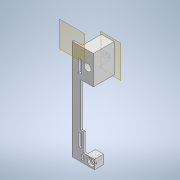
# Autodesk Inventor part: Display_Cover
Saved by Autodesk Inventor 2021 (Build 250183000, 183)
## iProperties
Created: 2020-08-10
Part Number: Display_Cover
Material: Generic
Document SubType Name: Modeling
Designer: ridvansong
Density: 1 g/cm^3
Appearance: Default
Author: ridvansong
Autodesk Inventor part; units mm, degrees
ref_plane "YZ Plane" through (0, 0, 0) normal (1, 0, 0) x (0, 1, 0)
ref_plane "XZ Plane" through (0, 0, 0) normal (0, 1, 0) x (-1, 0, 0)
ref_plane "XY Plane" through (0, 0, 0) normal (0, 0, 1) x (1, 0, 0)
ref_plane "Work Plane1" through (0, 0, 0) normal (0, 0, 1) x (1, 0, 0)
sketch "Sketch1" plane through (0, 0, 0) normal (0, 0, 1) x (1, 0, 0)
  line L0 (11.775, 18.625) -> (-4.025, 18.625) projected
  line L1 (11.775, 43.875) -> (11.775, 18.625) projected
  line L2 (-4.025, 43.875) -> (11.775, 43.875) projected
  line L3 (-4.025, 18.625) -> (-4.025, 43.875) projected
  line L4 (7.775, 43.875) -> (7.775, -42.625) projected
  line L5 (-4.025, 18.625) -> (6.775, 18.625)
  line L6 (6.775, 18.625) -> (6.775, 43.375)
  line L7 (6.775, 43.375) -> (-4.025, 43.375)
  line L8 (-4.025, 43.375) -> (-4.025, 18.625)
  circle A0 centre (1.775, 30.625) radius 1.3 projected
  line L9 (11.775, -42.625) -> (11.775, -34.625) projected
  line L10 (11.775, -34.625) -> (2.775, -34.625) projected
  line L11 (2.775, -34.625) -> (2.775, -42.625) projected
  line L12 (11.775, -42.625) -> (2.775, -42.625) projected
  line L13 (7.275, -34.625) -> (0.775, -34.625)
  line L14 (0.775, -34.625) -> (0.775, -42.125)
  line L15 (0.775, -42.125) -> (7.275, -42.125)
  line L16 (7.275, -42.125) -> (7.275, -34.625)
  circle A1 centre (4.775, -38.375) radius 1.3 projected
  point P0 (0, 0)
  point P1 (-4.025, 43.375)
  dimension "d0" = 0.5
  dimension "d1" = 1
  dimension "d30" = 0.5
  dimension "d31" = 6.5
  constraints: 16 end point, 4 parallel, 2 collinear, 2 horizontal, 2 perpendicular, 1 midpoint
  measures "d0" distance between parallel lines of L2 L7
  measures "d1" distance between parallel lines of L4 L6
  measures "d30" distance between parallel lines of L15 L12
  measures "d31" distance between parallel lines of L16 L14
ref_plane "Work Plane2" through (-11.525, -42.375, 16.25) normal (0, 0, 1) x (1, 0, 0)
extrude "Extrusion1" add sketch "Sketch1" along normal up to surface (16.25 mm away) contours L0 L3 L7 L6
sketch "Sketch2" plane through (-4.025, 43.375, 16.25) normal (0, 0, 1) x (1, 0, 0)
  line L0 (-7.5, -85.75) -> (-7.5, 0)
  line L1 (-7.5, 0) -> (10.8, 0)
  line L2 (10.8, -24.75) -> (10.8, 0) projected
  line L3 (10.8, 0) -> (10.8, -24.75)
  line L4 (0, -24.75) -> (10.8, -24.75) projected
  line L5 (10.8, -24.75) -> (0, -24.75)
  line L6 (0, -24.75) -> (0, -64.5)
  line L7 (0, -64.5) -> (-1.85, -64.5)
  line L8 (-1.85, -64.5) -> (-1.85, -75.5)
  line L9 (-1.85, -75.5) -> (0, -75.5)
  line L10 (-7.5, -85.75) -> (6.5, -85.75) projected
  line L11 (-7.5, 0.25) -> (-7.5, -85.75) projected
  line L12 (0, -64.75) -> (0, -75.25) projected
  line L13 (0, -64.75) -> (-1.6, -64.75) projected
  line L14 (-1.6, -75.25) -> (-1.6, -64.75) projected
  line L15 (0, -75.25) -> (-1.6, -75.25) projected
  line L16 (0, -9.75) -> (0, -20.25) projected
  line L17 (0, -9.75) -> (-1.6, -9.75) projected
  line L18 (-1.6, -20.25) -> (-1.6, -9.75) projected
  line L19 (0, -20.25) -> (-1.6, -20.25) projected
  line L20 (-1.85, -9.5) -> (0.25, -9.5)
  line L21 (0.25, -9.5) -> (0.25, -20.5)
  line L22 (0.25, -20.5) -> (-1.85, -20.5)
  line L23 (-1.85, -20.5) -> (-1.85, -9.5)
  line L24 (0, 0) -> (10.8, 0) projected
  line L25 (15.8, -86) -> (15.8, -78) projected
  line L26 (15.8, -78) -> (6.8, -78) projected
  line L27 (6.8, -78) -> (6.8, -86) projected
  line L28 (15.8, -86) -> (6.8, -86) projected
  line L29 (11.8, -217.75) -> (11.8, 42.25)
  line L30 (11.8, -85.75) -> (11.8, -78)
  line L31 (11.8, -78) -> (0, -78)
  line L32 (0, -78) -> (0, -75.5)
  line L33 (-7.5, -85.75) -> (11.8, -85.75)
  line L34 (0.5, -83.875) -> (0.5, -79.875)
  line L35 (0.5, -79.875) -> (2, -79.875)
  line L36 (2, -79.875) -> (2, -83.875)
  line L37 (2, -83.875) -> (0.5, -83.875)
  line L38 (0, -75.5) -> (0.25, -75.5)
  line L39 (0.25, -75.5) -> (0.25, -64.5)
  line L40 (0.25, -64.5) -> (0, -64.5)
  line L41 (2.25, -78) -> (2.25, -62.5)
  line L42 (2.25, -62.5) -> (0, -62.5)
  circle A0 centre (8.8, -81.75) radius 1.3 projected
  point P0 (4.025, -43.375)
  point P1 (-7.5, -85.75)
  point P2 (6.5, -85.75)
  point P3 (6.8, -85.75)
  dimension "d4" = 0.25
  dimension "d5" = 0.25
  dimension "d6" = 0.25
  dimension "d7" = 0.25
  dimension "d22" = 4
  dimension "d23" = 1.875
  dimension "d24" = 1.5
  dimension "d25" = 8
  dimension "d44" = 0.25
  dimension "d45" = 2
  dimension "d46" = 2
  constraints: 52 end point, 13 perpendicular, 7 point on line, 4 collinear, 3 vertical, 1 horizontal, 5 other
  measures "d4" distance between parallel lines of L18 L23
  measures "d5" distance between parallel lines of L8 L14
  measures "d6" distance between parallel lines of L13 L7
  measures "d7" distance between parallel lines of L15 L9
  measures "d22" distance of L34.start L34.end
  measures "d23" distance between parallel lines of L33 L37
  measures "d24" distance between parallel lines of L36 L34
  measures "d25" distance between parallel lines of L0 L34
  measures "d44" distance between parallel lines of L12 L39
  measures "d45" distance between parallel lines of L7 L42
  measures "d46" distance between parallel lines of L41 L39
ref_plane "Work Plane3" through (-12.525, -42.875, 17.75) normal (0, 0, 1) x (1, 0, 0)
ref_plane "Work Plane4" through (-11.525, 43.375, 17.75) normal (0, 0, 1) x (1, 0, 0)
ref_plane "Work Plane5" through (-12.525, -42.875, 17.75) normal (0, 0, 1) x (1, 0, 0)
extrude "Extrusion3" add sketch "Sketch2" along normal up to surface (1.5 mm away) contours L0 L1 L2 L4 L6 L7 L8 L9 L32 L31 L27 L33 L10 | L27 L26 L29 L33 | L31 L32 L38 L39 L40 L6 L42 L41 | A0
sketch "Sketch3" plane through (-11.525, 43.375, 17.75) normal (0, 0, 1) x (1, 0, 0)
  line L0 (18.3, 0) -> (18.3, -24.75) projected
  line L1 (18.3, -24.75) -> (7.5, -24.75) projected
  line L2 (14.3, -78) -> (14.3, -86) projected
  line L3 (9.75, -78) -> (19.3, -78) projected
  point P0 (11.525, -43.375)
  point P1 (13.3, -12.75)
  point P2 (7.5, -78)
  dimension "d13" = 5
  dimension "d14" = 12
  measures "d13" distance from line of L0 point (13.3, -12.75)
  measures "d14" distance from line of L1 point (13.3, -12.75)
hole "Hole1" at (1.775, 30.625, 17.75) direction (0, 0, -1) diameter 3.2 end through all counterbore diameter 6 counterbore depth 16.5
sketch "Sketch4" plane through (-4.025, 43.375, 16.25) normal (0, 0, -1) x (-1, 0, 0)
  line L0 (-2.25, -78) -> (-11.8, -78) projected
  line L1 (-11.8, -78) -> (-11.8, -85.75) projected
  line L2 (-4.8, -78) -> (-11.8, -78)
  line L3 (-11.8, -78) -> (-11.8, -85.75)
  line L4 (-11.8, -85.75) -> (-4.8, -85.75)
  line L5 (-4.8, -85.75) -> (-4.8, -78)
  point P0 (-4.025, -43.375)
  point P1 (0, -78)
  dimension "d32" = 7
  constraints: 8 end point, 2 parallel, 1 horizontal, 1 perpendicular, 1 point on line
  measures "d32" distance between parallel lines of L1 L5
ref_plane "Work Plane6" through (2.775, -42.625, 10) normal (0, 0, 1) x (1, 0, 0)
extrude "Extrusion4" add sketch "Sketch4" along normal up to surface (6.25 mm away)
sketch "Sketch5" plane through (-11.525, -42.375, 17.75) normal (0, 0, 1) x (1, 0, 0)
  line L0 (19.3, 7.75) -> (19.3, 0) projected
  line L1 (9.75, 7.75) -> (19.3, 7.75) projected
  point P0 (11.525, 42.375)
  point P1 (16.3, 4)
  point P2 (7.5, 7.75)
  dimension "d35" = 3
  dimension "d36" = 3.75
  measures "d35" distance from line of point (16.3, 4) L0
  measures "d36" distance from line of L1 point (16.3, 4)
hole "Hole2" at (4.775, -38.375, 17.75) direction (0, 0, -1) diameter 3.2 end through all counterbore diameter 6 counterbore depth 2
body "Solid1"
